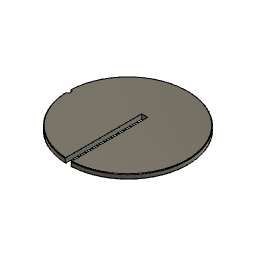
JetBandSawThroatPlate v1 (Autodesk Fusion 360 design; units mm, degrees)
Autodesk Fusion 360 part; units mm, degrees
sketch "Sketch1" plane through (0, 0, 0) normal (0, 1, 0) x (1, 0, 0)
  circle A0 centre (0, 0) radius 31.8135
  line L0 (0, 0) -> (-1.5875, 0) construction
  line L1 (-1.5875, 0) -> (-1.5875, -31.7739)
  line L2 (1.5875, 0) -> (1.5875, -31.7739)
  line L3 (-1.5875, 0) -> (-1.5875, 8.89)
  line L4 (-1.5875, 8.89) -> (1.5875, 8.89)
  line L5 (1.5875, 8.89) -> (1.5875, 0)
  line L6 (0, 0) -> (-31.8135, 0) construction
  circle A1 centre (-31.8135, 0) radius 1.5
  dimension "d1" = 63.627
  dimension "d2" = 1.5875
  dimension "d3" = 3.175
  dimension "d4" = 8.89
  dimension "d5" = 3.175
  dimension "d10" = 3
  constraint coincident A0.centre L0.start
  constraint horizontal L0
  constraint coincident A0 L1.end
  constraint coincident A0 L2.end
  constraint perpendicular L0 L3
  constraint perpendicular L3 L4
  constraint perpendicular L4 L5
  constraint coincident A0 L6.end
  constraint perpendicular L2 L6
  constraint coincident L6.end A1.centre
  measures "d1" diameter of A0
  measures "d2" distance of A0.centre L0.end
  measures "d3" distance of L0.end L2.start
  measures "d4" distance of L0.end L3.end
  measures "d5" distance of L3.end L4.end
  measures "d10" diameter of A1
extrude "Extrude1" add sketch "Sketch1" along normal blind 2.4892 contours A0 L1 L2 L3 L4 L5 A1 | A0 A1 picked at (-31.3109, 0) in component "Component"
fillet "Fillet1" radius 0.254 1 edges at (0, 2.4892, -31.8135) in component "Component"
fillet "Fillet2" radius 0.254 1 edges at (0, 0, -31.8135) in component "Component"
extrude "Extrude2" cut sketch "Sketch1" along normal up to surface (2.4892 mm away) contours A0 A1 picked at (-31.3109, 0) in component "Component"
component "Component" placed x (1, 0, 0) y (0, 1, 0) z (0, 0, 1) at (0, 0, 0)
equation "d2 = ( 0.125 / 2 ) * 1 in"
